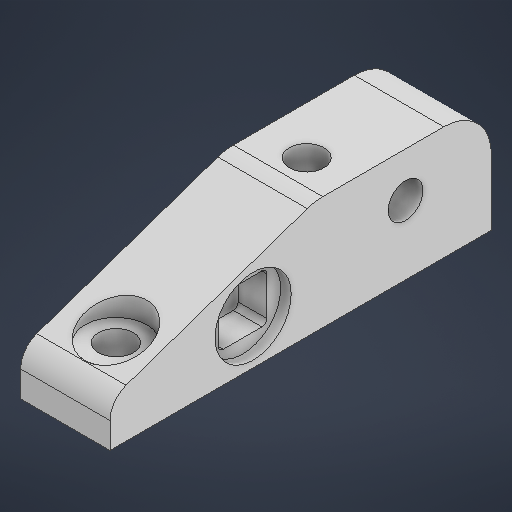
# Autodesk Inventor part: Pass_Hang_Block
Saved by Autodesk Inventor 2025.1 (Build 291241000, 241)
## iProperties
Created: 2025-01-10
Part Number: Pass_Hang_Block
Material: Generic
Document SubType Name: Modeling
Designer: Juanl
Density: 1 g/cm^3
Appearance: Default
Author: Juanl
Autodesk Inventor part; units mm, degrees
ref_plane "YZ Plane" through (0, 0, 0) normal (1, 0, 0) x (0, 1, 0)
ref_plane "XZ Plane" through (0, 0, 0) normal (0, 1, 0) x (-1, 0, 0)
ref_plane "XY Plane" through (0, 0, 0) normal (0, 0, 1) x (1, 0, 0)
sketch "Sketch1" plane through (0, 0, 0) normal (1, 0, 0) x (0, 1, 0)
  line L0 (-1.51927, 9.235223) -> (-1.51927, -28.864777)
  circle A0 centre (4.445248, -9.814777) radius 2.1844
  circle A1 centre (4.445248, -9.814777) radius 5.964518
  line L1 (4.445248, -9.814777) -> (-1.51927, -9.814777)
  line L2 (-1.51927, -9.814777) -> (-1.51927, 9.235223)
  line L3 (-1.51927, 9.235223) -> (-1.51927, -28.864777)
  line L4 (-1.51927, 9.235223) -> (1.02073, 9.235223)
  line L5 (1.02073, 9.235223) -> (9.344761, -6.41327)
  line L6 (-1.51927, -28.864777) -> (1.02073, -28.864777)
  line L7 (1.02073, -28.864777) -> (9.344761, -13.216284)
  point P0 (0, 0)
  dimension "d0" = 5.96452
  dimension "d1" = 19.05
  dimension "d2" = 38.1
  dimension "d3" = 2.54
  constraints: 16 end point, 3 point on circle, 2 centre point, 2 horizontal, 1 coincident, 1 midpoint, 1 tangent
  measures "d0" distance from line of L0 A0.centre
  measures "d1" distance of L0.start L1.end
  measures "d2" distance of L0.start L0.end
  measures "d3" distance of L0.start L4.end
extrude "Extrusion1" add sketch "Sketch1" along normal blind 11.9126
sketch "Sketch2" plane through (0, -1.51927, -28.864777) normal (0, -1, 0) x (1, 0, 0)
  line L0 (0, 38.1) -> (0, 0) projected
  line L1 (0, 0) -> (11.9126, 0) projected
  line L2 (11.9126, 38.1) -> (11.9126, 0) projected
  line L3 (0, 38.1) -> (11.9126, 38.1) projected
  line L4 (0, 38.1) -> (6.35, 38.1)
  line L5 (6.35, 38.1) -> (6.35, 0)
  line L6 (6.35, 38.1) -> (6.35, 31.75)
  line L7 (6.35, 31.75) -> (6.35, 6.35)
  line L8 (6.35, 6.35) -> (6.35, 0)
  circle A0 centre (6.35, 31.75) radius 2.3241
  circle A1 centre (6.35, 6.35) radius 2.3241
  circle A2 centre (6.35, 19.05) radius 2.2225
  point P0 (0, 28.864777)
  dimension "d6" = 6.35
  dimension "d7" = 6.35
  dimension "d8" = 25.4
  dimension "d9" = 4.6482
  dimension "d10" = 4.445
  constraints: 10 end point, 4 point on line, 3 centre point, 2 coincident, 1 collinear, 1 midpoint, 1 perpendicular
  measures "d6" distance of L0.start L4.end
  measures "d7" distance of L4.end L6.end
  measures "d8" distance of L6.end L7.end
  measures "d9" diameter of A0
  measures "d10" diameter of A2
extrude "Extrusion2" cut sketch "Sketch2" against normal through all contours A0 L5 | L5 A0 | A1 L5 | L5 A1
sketch "Sketch3" plane through (11.9126, 0, 0) normal (1, 0, 0) x (0, 0, -1)
  line L0 (28.864777, -1.51927) -> (28.864777, 1.02073)
  line L1 (28.864777, 1.02073) -> (13.216284, 9.344761)
  arc A0 (13.216284, 9.344761) -> (6.41327, 9.344761) centre (9.814777, 4.445248) ccw
  line L2 (6.41327, 9.344761) -> (-9.235223, 1.02073)
  line L3 (-9.235223, 1.02073) -> (-9.235223, -1.51927)
  line L4 (-9.235223, -1.51927) -> (28.864777, -1.51927)
  circle A1 centre (9.814777, 4.445248) radius 2.1844
  line L5 (9.814777, 10.409766) -> (28.864777, 10.409766)
  line L6 (28.864777, 10.409766) -> (28.864777, -1.51927)
  line L7 (20.190677, 5.634815) -> (24.838877, 3.16226)
  line L8 (24.838877, -1.51927) -> (20.190677, -1.51927)
  line L9 (22.514777, -1.51927) -> (22.514777, 10.409766)
  line L10 (22.514777, 10.409766) -> (35.214777, 10.409766)
  line L11 (35.214777, 10.409766) -> (35.214777, -1.51927)
  line L12 (35.214777, -1.51927) -> (28.864777, -1.51927)
  line L13 (-9.235223, 1.02073) -> (-9.235223, 4.19573)
  line L14 (-9.235223, 4.19573) -> (7.873428, 10.084986)
  point P0 (0, 0)
  dimension "d13" = 12.7
  dimension "d14" = 3.175
  constraints: 16 end point, 4 perpendicular, 2 horizontal, 2 point on circle, 1 midpoint, 1 point on line, 1 tangent, 1 vertical
  measures "d13" distance of L9.end L10.end
  measures "d14" distance of L2.end L13.end
extrude "Extrusion3" add sketch "Sketch3" against normal up to surface (11.9126 mm away) contours L0 L6 L10 L11 L12 | L1 L9 L5 L6 | L1 A0 L5 L9 | A0 L2 L13 L14
sketch "Sketch4" plane through (0, -1.51927, 9.235223) normal (0, -1, 0) x (1, 0, 0)
  circle A0 centre (6.35, -31.75) radius 2.3241 projected
  circle A1 centre (6.35, -6.35) radius 2.3241 projected
  line L0 (0, 0) -> (0, -44.45) projected
  line L1 (11.9126, -44.45) -> (0, -44.45) projected
  line L2 (11.9126, 0) -> (11.9126, -44.45) projected
  line L3 (0, 0) -> (11.9126, 0) projected
  point P0 (0, -9.235223)
extrude "Extrusion4" cut sketch "Sketch4" against normal through all contours A0 | A1
sketch "Sketch6" plane through (0, -1.51927, 9.235223) normal (0, -1, 0) x (1, 0, 0)
  line L0 (11.9126, -16.8656) -> (0, -16.8656) projected
  circle A0 centre (6.35, -31.75) radius 2.3241 projected
  circle A1 centre (6.35, -6.35) radius 2.3241 projected
  line L1 (0, 0) -> (0, -44.45) projected
  line L2 (11.9126, -44.45) -> (0, -44.45) projected
  line L3 (11.9126, 0) -> (11.9126, -44.45) projected
  line L4 (0, 0) -> (11.9126, 0) projected
  line L5 (6.35, -6.35) -> (6.35, -19.05)
  circle A2 centre (6.35, -19.05) radius 2.2225
  line L6 (7.3025, -16.8275) -> (5.3975, -16.8275)
  line L7 (4.1275, -18.0975) -> (4.1275, -20.0025)
  line L8 (5.3975, -21.2725) -> (7.3025, -21.2725)
  line L9 (8.5725, -20.0025) -> (8.5725, -18.0975)
  arc A3 (8.5725, -18.0975) -> (7.3025, -16.8275) centre (7.3025, -18.0975) ccw
  arc A4 (7.3025, -21.2725) -> (8.5725, -20.0025) centre (7.3025, -20.0025) ccw
  arc A5 (5.3975, -16.8275) -> (4.1275, -18.0975) centre (5.3975, -18.0975) ccw
  arc A6 (4.1275, -20.0025) -> (5.3975, -21.2725) centre (5.3975, -20.0025) ccw
  point P0 (0, -9.235223)
  dimension "d20" = 12.7
  dimension "d21" = 4.445
  dimension "d22" = 1.27
  constraints: 10 end point, 8 point on circle, 8 tangent, 5 centre point, 3 equal radius, 2 parallel, 1 coincident, 1 horizontal, 1 perpendicular, 1 vertical
  measures "d20" distance of L5.start L5.end
  measures "d21" diameter of A2
  measures "d22" radius of A3
sketch "Sketch6 outline for Extrusion5" plane through (0, -1.51927, 9.235223) normal (0, -1, 0) x (1, 0, 0)
  arc A0 (4.1275, -20.0025) -> (5.3975, -21.2725) centre (5.3975, -20.0025) ccw
  line L0 (4.1275, -18.0975) -> (4.1275, -20.0025)
  arc A1 (5.3975, -16.8275) -> (4.1275, -18.0975) centre (5.3975, -18.0975) ccw
  line L1 (7.3025, -16.8275) -> (5.3975, -16.8275)
  arc A2 (8.5725, -18.0975) -> (7.3025, -16.8275) centre (7.3025, -18.0975) ccw
  line L2 (8.5725, -20.0025) -> (8.5725, -18.0975)
  arc A3 (7.3025, -21.2725) -> (8.5725, -20.0025) centre (7.3025, -20.0025) ccw
  line L3 (5.3975, -21.2725) -> (7.3025, -21.2725)
extrude "Extrusion5" add sketch "Sketch6 outline for Extrusion5" along normal blind 1.6002
sketch "Sketch7" plane through (0, -1.51927, 9.235223) normal (0, -1, 0) x (1, 0, 0)
  arc A0 (4.1275, -20.0025) -> (5.3975, -21.2725) centre (5.3975, -20.0025) ccw projected
  line L0 (4.1275, -20.0025) -> (4.1275, -18.0975) projected
  arc A1 (5.3975, -16.8275) -> (4.1275, -18.0975) centre (5.3975, -18.0975) ccw projected
  line L1 (5.3975, -16.8275) -> (7.3025, -16.8275) projected
  arc A2 (8.5725, -18.0975) -> (7.3025, -16.8275) centre (7.3025, -18.0975) ccw projected
  line L2 (8.5725, -18.0975) -> (8.5725, -20.0025) projected
  arc A3 (7.3025, -21.2725) -> (8.5725, -20.0025) centre (7.3025, -20.0025) ccw projected
  line L3 (7.3025, -21.2725) -> (5.3975, -21.2725) projected
  circle A4 centre (6.35, -31.75) radius 2.3241 projected
  circle A5 centre (6.35, -6.35) radius 2.3241 projected
  line L4 (0, 0) -> (0, -44.45) projected
  line L5 (11.9126, -44.45) -> (0, -44.45) projected
  line L6 (11.9126, 0) -> (11.9126, -44.45) projected
  line L7 (0, 0) -> (11.9126, 0) projected
  line L8 (11.9126, -44.45) -> (11.9126, -50.8)
  line L9 (11.9126, 0) -> (11.9126, -44.45) projected
  line L10 (11.9126, -50.8) -> (0, -50.8)
  line L11 (0, -50.8) -> (0, -44.45)
  line L12 (6.35, -31.75) -> (6.35, -44.45)
  circle A6 centre (6.35, -44.45) radius 2.2225
  line L13 (7.3025, -42.2275) -> (5.3975, -42.2275)
  line L14 (4.1275, -43.4975) -> (4.1275, -45.4025)
  line L15 (5.3975, -46.6725) -> (7.3025, -46.6725)
  line L16 (8.5725, -45.4025) -> (8.5725, -43.4975)
  arc A7 (8.5725, -43.4975) -> (7.3025, -42.2275) centre (7.3025, -43.4975) ccw
  arc A8 (7.3025, -46.6725) -> (8.5725, -45.4025) centre (7.3025, -45.4025) ccw
  arc A9 (4.1275, -45.4025) -> (5.3975, -46.6725) centre (5.3975, -45.4025) ccw
  arc A10 (5.3975, -42.2275) -> (4.1275, -43.4975) centre (5.3975, -43.4975) ccw
  point P0 (0, -9.235223)
  dimension "d25" = 6.35
  dimension "d26" = 12.7
  dimension "d27" = 4.445
  dimension "d28" = 1.27
  constraints: 16 end point, 8 point on circle, 8 tangent, 5 centre point, 3 equal radius, 3 perpendicular, 2 parallel, 1 coincident, 1 collinear, 1 horizontal, 1 point on line
  measures "d25" distance of L5.start L8.end
  measures "d26" distance of L12.start L12.end
  measures "d27" diameter of A6
  measures "d28" radius of A7
extrude "Extrusion6" add sketch "Sketch7" against normal up to surface (11.929036 mm away) contours L5 L14 A9 L15 A8 L16 L8 L10 L11 | L5 A6 | A6 L15 A9 L14 | A6 L16 A8 L15
extrude "Extrusion7" add sketch "Sketch7" along normal blind 1.6002 contours A6 L12 L5 | L14 A10 L13 A6 | L5 A6 | A6 L15 A9 L14 | L12 A6 L5 | L13 A7 L16 A6 | A6 L16 A8 L15
sketch "Sketch8" plane through (11.9126, 0, 0) normal (1, 0, 0) x (0, 0, -1)
  line L0 (24.838877, -1.51927) -> (24.838877, 10.409766)
  arc A0 (9.814777, 10.409766) -> (7.873428, 10.084986) centre (9.814777, 4.445248) ccw
  line L1 (7.873428, 10.084986) -> (-9.235223, 4.19573)
  line L2 (-9.235223, 4.19573) -> (-9.235223, -1.51927)
  line L3 (-9.235223, -1.51927) -> (41.564777, -1.51927)
  line L4 (41.564777, -1.51927) -> (41.564777, 10.409766)
  line L5 (41.564777, 10.409766) -> (9.814777, 10.409766)
  circle A1 centre (9.814777, 4.445248) radius 2.1844
  line L6 (-9.235223, 4.19573) -> (18.040506, 13.584766)
  line L7 (14.316656, 13.584766) -> (41.564777, 13.584766)
  line L8 (41.564777, 13.584766) -> (41.564777, 10.409766)
  point P0 (0, 0)
  point P1 (7.873428, 10.084986)
  constraints: 6 end point, 1 horizontal, 1 perpendicular, 1 point on line
extrude "Extrusion8" add sketch "Sketch8" against normal up to surface (11.9126 mm away) contours L5 A0 L6 L7 L8
sketch "Sketch9" plane through (11.9126, 0, 0) normal (1, 0, 0) x (0, 0, -1)
  line L0 (18.040506, 13.584766) -> (-9.235223, 4.19573)
  line L1 (-9.235223, 4.19573) -> (-9.235223, -1.51927)
  line L2 (-9.235223, -1.51927) -> (41.564777, -1.51927)
  line L3 (41.564777, -1.51927) -> (41.564777, 13.584766)
  line L4 (41.564777, 13.584766) -> (18.040506, 13.584766)
  circle A0 centre (9.814777, 4.445248) radius 2.1844
  line L5 (9.814777, 4.445248) -> (35.214777, 4.445248)
  line L6 (35.214777, 4.445248) -> (35.214777, 7.620248)
  circle A1 centre (35.214777, 7.620248) radius 2.3241
  circle A2 centre (35.214777, 7.620248) radius 5.08
  line L7 (35.214777, 7.620248) -> (30.134777, 7.620248)
  circle A3 centre (30.134777, 7.620248) radius 2.3241
  point P0 (0, 0)
  dimension "d36" = 25.4
  dimension "d37" = 3.175
  dimension "d38" = 4.6482
  dimension "d49" = 10.16
  dimension "d57" = 5.08
  dimension "d58" = 4.6482
  constraints: 6 end point, 3 centre point, 3 coincident, 2 horizontal, 1 perpendicular
  measures "d36" distance of L5.start L5.end
  measures "d37" distance of L5.end L6.end
  measures "d38" diameter of A1
  measures "d49" diameter of A2
  measures "d57" distance of L7.start L7.end
  measures "d58" diameter of A3
fillet "Fillet1" radius 3.175 1 edges at (5.9563, 4.1957, 9.2352)
sketch "Sketch10" plane through (11.9126, 0, 0) normal (1, 0, 0) x (0, 0, -1)
  line L0 (-5.209323, 5.581553) -> (-0.561123, 7.181587)
  line L1 (-0.561123, -1.51927) -> (-5.209323, -1.51927)
  line L2 (-2.885223, 6.38157) -> (-0.561123, 6.38157)
  line L3 (-0.561123, -1.51927) -> (-0.561123, 7.181587)
  line L4 (-0.561123, 6.38157) -> (-5.209323, 6.38157)
  line L5 (-5.209323, -1.51927) -> (-5.209323, 5.581553)
  line L6 (-0.561123, 6.38157) -> (-0.561123, 8.069179)
  line L7 (-0.561123, 8.069179) -> (-5.209323, 8.069179)
  line L8 (-5.209323, 8.069179) -> (-5.209323, 5.581553)
  point P0 (0, 0)
  constraints: 10 end point, 3 perpendicular, 2 point on line, 1 horizontal, 1 midpoint, 1 vertical
extrude "Extrusion9" add sketch "Sketch10" against normal up to surface (11.9126 mm away) contours L8 L4 L0 | L4 L8 L7 L6 L0
sketch "Sketch11" plane through (11.9126, 8.069179, 5.209323) normal (0, 1, 0) x (1, 0, 0)
  arc A0 (-5.5626, 4.6482) -> (-5.5626, 0) centre (-5.5626, 2.3241) ccw projected
  arc A1 (-5.5626, 0) -> (-5.5626, 4.6482) centre (-5.5626, 2.3241) ccw projected
  circle A2 centre (-5.5626, 2.3241) radius 2.3241 projected
  arc A3 (-5.5626, 4.6482) -> (-5.5626, 0) centre (-5.5626, 2.3241) ccw projected
  circle A4 centre (-5.5626, 2.3241) radius 4.1275
  point P0 (-11.9126, 5.209323)
  dimension "d42" = 8.255
  constraints: 1 centre point, 1 coincident
  measures "d42" diameter of A4
extrude "Extrusion10" cut sketch "Sketch11" against normal blind 3.1115 contours A1 A0 | A4
sketch "Sketch12" plane through (11.9126, 0, 0) normal (1, 0, 0) x (0, 0, -1)
  circle A0 centre (9.814777, 4.445248) radius 2.1844
  arc A1 (-7.093632, 4.932923) -> (-9.235223, 1.930809) centre (-6.060223, 1.930809) ccw
  line L0 (-9.235223, 1.930809) -> (-9.235223, -1.51927)
  line L1 (-9.235223, -1.51927) -> (41.564777, -1.51927)
  line L2 (41.564777, -1.51927) -> (41.564777, 13.584766)
  line L3 (41.564777, 13.584766) -> (18.040506, 13.584766)
  line L4 (18.040506, 13.584766) -> (-0.561123, 7.181587)
  line L5 (-0.561123, 7.181587) -> (-0.561123, 8.069179)
  line L6 (-0.561123, 8.069179) -> (-5.209323, 8.069179)
  line L7 (-5.209323, 8.069179) -> (-5.209323, 5.581553)
  line L8 (-5.209323, 5.581553) -> (-7.093632, 4.932923)
  line L9 (-5.209323, 5.581553) -> (-0.561123, 7.181587)
  point P0 (0, 0)
  constraints: 2 end point, 1 collinear
extrude "Extrusion11" cut sketch "Sketch12" along normal through all both and the other way through all contours L7 L6 L5 L9
sketch "Sketch13" plane through (0, -1.51927, 9.235223) normal (0, -1, 0) x (1, 0, 0)
  circle A0 centre (6.35, -6.35) radius 4.1275 projected
  arc A1 (5.3975, -42.2275) -> (4.1275, -43.4975) centre (5.3975, -43.4975) ccw projected
  line L0 (5.3975, -42.2275) -> (7.3025, -42.2275) projected
  arc A2 (8.5725, -43.4975) -> (7.3025, -42.2275) centre (7.3025, -43.4975) ccw projected
  line L1 (8.5725, -43.4975) -> (8.5725, -45.4025) projected
  arc A3 (7.3025, -46.6725) -> (8.5725, -45.4025) centre (7.3025, -45.4025) ccw projected
  line L2 (7.3025, -46.6725) -> (5.3975, -46.6725) projected
  arc A4 (4.1275, -45.4025) -> (5.3975, -46.6725) centre (5.3975, -45.4025) ccw projected
  line L3 (4.1275, -45.4025) -> (4.1275, -43.4975) projected
  arc A5 (4.1275, -20.0025) -> (5.3975, -21.2725) centre (5.3975, -20.0025) ccw projected
  line L4 (4.1275, -20.0025) -> (4.1275, -18.0975) projected
  arc A6 (5.3975, -16.8275) -> (4.1275, -18.0975) centre (5.3975, -18.0975) ccw projected
  line L5 (5.3975, -16.8275) -> (7.3025, -16.8275) projected
  arc A7 (8.5725, -18.0975) -> (7.3025, -16.8275) centre (7.3025, -18.0975) ccw projected
  line L6 (8.5725, -18.0975) -> (8.5725, -20.0025) projected
  arc A8 (7.3025, -21.2725) -> (8.5725, -20.0025) centre (7.3025, -20.0025) ccw projected
  line L7 (7.3025, -21.2725) -> (5.3975, -21.2725) projected
  circle A9 centre (6.35, -31.75) radius 2.3241 projected
  circle A10 centre (6.35, -6.35) radius 2.3241 projected
  line L8 (0, 0) -> (0, -50.8) projected
  line L9 (0, -50.8) -> (11.9126, -50.8) projected
  line L10 (11.9126, 0) -> (11.9126, -50.8) projected
  line L11 (0, 0) -> (11.9126, 0) projected
  point P0 (0, -9.235223)
extrude "Extrusion12" cut sketch "Sketch13" along normal through all both and the other way through all contours A9
extrude "Extrusion13" [suppressed]
sketch "Sketch14" plane through (11.9126, 0, 0) normal (1, 0, 0) x (0, 0, -1)
  line L0 (18.040506, 13.584766) -> (-7.093632, 4.932923)
  arc A0 (-7.093632, 4.932923) -> (-9.235223, 1.930809) centre (-6.060223, 1.930809) ccw
  line L1 (-9.235223, 1.930809) -> (-9.235223, -1.51927)
  line L2 (-9.235223, -1.51927) -> (41.564777, -1.51927)
  line L3 (41.564777, -1.51927) -> (41.564777, 13.584766)
  line L4 (41.564777, 13.584766) -> (18.040506, 13.584766)
  circle A1 centre (9.814777, 4.445248) radius 2.1844
  circle A2 centre (9.814777, 4.445248) radius 5.08
  point P0 (0, 0)
  dimension "d52" = 10.16
  constraints: 1 centre point, 1 coincident
  measures "d52" diameter of A2
extrude "Extrusion14" cut sketch "Sketch14" against normal blind 1.397 contours A2
sketch "Sketch15" plane through (10.5156, 4.445248, -9.814777) normal (1, 0, 0) x (0, 0, -1)
  line L0 (-3.22834, 2.577465) -> (-3.22834, -2.577465)
  circle A0 centre (0, 0) radius 2.032
  line L1 (-2.577465, -3.22834) -> (2.577465, -3.22834)
  arc A1 (-3.22834, -2.577465) -> (-2.577465, -3.22834) centre (-2.577465, -2.577465) ccw
  arc A2 (-2.577465, 3.22834) -> (-3.22834, 2.577465) centre (-2.577465, 2.577465) ccw
  line L2 (2.577465, 3.22834) -> (-2.577465, 3.22834)
  arc A3 (3.22834, 2.577465) -> (2.577465, 3.22834) centre (2.577465, 2.577465) ccw
  line L3 (3.22834, -2.577465) -> (3.22834, 2.577465)
  arc A4 (2.577465, -3.22834) -> (3.22834, -2.577465) centre (2.577465, -2.577465) ccw
  circle A5 centre (0, 0) radius 5.08
  circle A6 centre (0, 0) radius 2.1844
  point P0 (-9.814777, -4.445248)
  constraints: 8 end point, 8 point on circle, 5 centre point
extrude "Extrusion15" cut sketch "Sketch15" against normal blind 3.81 contours A2 L2 A3 L3 A4 L1 A1 L0
extrude "Extrusion16" cut sketch "Sketch9" along normal through all both and the other way through all contours A3 A2 | A2 L7 A3 | A2 A3 L7
fillet "Fillet2" radius 6.35 1 edges at (5.9563, 13.5848, -18.0405)
fillet "Fillet3" radius 6.35 1 edges at (5.9563, 13.5848, -41.5648)
body "Solid1"
